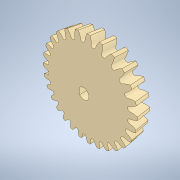
# Autodesk Inventor part: Шестерня мотора 2
Saved by Autodesk Inventor 2021.1 (Build 251245010, 245A)
## iProperties
Created: 2026-05-03
Part Number: Шестерня мотора 2
Material: Generic
Document SubType Name: Modeling
Designer: Андрей Тарасов
Density: 1 g/cm^3
Appearance: Default
Author: Андрей Тарасов
Autodesk Inventor part; units mm, degrees
ref_plane "YZ Plane" through (0, 0, 0) normal (1, 0, 0) x (0, 1, 0)
ref_plane "XZ Plane" through (0, 0, 0) normal (0, 1, 0) x (-1, 0, 0)
ref_plane "XY Plane" through (0, 0, 0) normal (0, 0, 1) x (1, 0, 0)
sketch "Sketch1" plane through (0, 0, 0) normal (0, 0, 1) x (1, 0, 0)
  spline S0 degree 3 poles (-1.8162, 21.8754) (-1.7746, 21.8042) (-1.6912, 21.6617) (-1.5738, 21.4438) (-1.4622, 21.2229) (-1.3577, 20.9985) (-1.2608, 20.7707) (-1.1726, 20.5395) (-1.094, 20.3047) (-1.0278, 20.0662) (-0.9752, 19.824) (-0.9571, 19.6181) (-0.9246, 19.4563) (-0.8956, 19.3359) (-0.8558, 19.2186) (-0.8088, 19.104) (-0.7488, 18.9955) (-0.6764, 18.8948) (-0.6025, 18.8222) (-0.5374, 18.7714) (-0.4841, 18.7397) (-0.4281, 18.7132) (-0.3698, 18.6922) (-0.3092, 18.6789) (-0.1857, 18.6689) (0, 18.6787) (0.1857, 18.6689) (0.3092, 18.6789) (0.3698, 18.6922) (0.4281, 18.7132) (0.4841, 18.7397) (0.5374, 18.7714) (0.6025, 18.8222) (0.6764, 18.8948) (0.7488, 18.9955) (0.8088, 19.104) (0.8558, 19.2186) (0.8956, 19.3359) (0.9246, 19.4563) (0.9571, 19.6181) (0.9752, 19.824) (1.0278, 20.0662) (1.094, 20.3047) (1.1726, 20.5395) (1.2608, 20.7707) (1.3577, 20.9985) (1.4622, 21.2229) (1.5738, 21.4438) (1.6912, 21.6617) (1.7746, 21.8042) (1.8162, 21.8754) knots 0 0 0 0 0.024749 0.049497 0.074246 0.098994 0.123742 0.14849 0.173237 0.197983 0.222726 0.247472 0.259846 0.272219 0.284591 0.296962 0.309334 0.321703 0.334061 0.340251 0.346439 0.35262 0.358805 0.364993 0.371173 0.39592 0.420667 0.426846 0.433034 0.439219 0.4454 0.451589 0.457778 0.470137 0.482506 0.494877 0.507248 0.51962 0.531993 0.544367 0.569113 0.593856 0.618602 0.643349 0.668097 0.692845 0.717593 0.742342 0.767091 0.791839 0.791839 0.791839 0.791839
  circle A0 centre (0, 0) radius 18.6744 construction
  circle A1 centre (0, 0) radius 19.7335 construction
  circle A2 centre (0, 0) radius 21 construction
  circle A3 centre (0, 0) radius 21.9506
  spline S1 degree 3 poles (-6.6384, 20.9228) (-6.5819, 20.8626) (-6.469, 20.7423) (-6.306, 20.556) (-6.1481, 20.3654) (-5.9963, 20.1699) (-5.8512, 19.9694) (-5.7136, 19.7636) (-5.5848, 19.5521) (-5.4672, 19.3344) (-5.362, 19.1099) (-5.2985, 18.9133) (-5.2309, 18.7627) (-5.1758, 18.6518) (-5.1109, 18.5464) (-5.0395, 18.4451) (-4.957, 18.3526) (-4.8639, 18.2705) (-4.7757, 18.2162) (-4.701, 18.1811) (-4.6419, 18.1621) (-4.5815, 18.1488) (-4.5199, 18.1413) (-4.4579, 18.1417) (-4.3352, 18.1595) (-4.1564, 18.2104) (-3.9732, 18.2422) (-3.855, 18.2794) (-3.7989, 18.3059) (-3.7467, 18.3393) (-3.698, 18.3775) (-3.6531, 18.4203) (-3.6009, 18.4843) (-3.5451, 18.5715) (-3.4968, 18.6859) (-3.4626, 18.805) (-3.4422, 18.9272) (-3.4295, 19.0504) (-3.428, 19.1742) (-3.4324, 19.3392) (-3.4605, 19.5439) (-3.4631, 19.7918) (-3.4516, 20.039) (-3.4273, 20.2854) (-3.3927, 20.5305) (-3.3489, 20.7742) (-3.297, 21.0162) (-3.2374, 21.2564) (-3.1714, 21.495) (-3.1218, 21.6524) (-3.0971, 21.7311) knots 0 0 0 0 0.024749 0.049497 0.074246 0.098994 0.123742 0.14849 0.173237 0.197983 0.222726 0.247472 0.259846 0.272219 0.284591 0.296962 0.309334 0.321703 0.334061 0.340251 0.346439 0.35262 0.358805 0.364993 0.371173 0.39592 0.420667 0.426846 0.433034 0.439219 0.4454 0.451589 0.457778 0.470137 0.482506 0.494877 0.507248 0.51962 0.531993 0.544367 0.569113 0.593856 0.618602 0.643349 0.668097 0.692845 0.717593 0.742342 0.767091 0.791839 0.791839 0.791839 0.791839
  spline S2 degree 3 poles (-11.1277, 18.921) (-11.0593, 18.8749) (-10.9224, 18.7828) (-10.7221, 18.6374) (-10.5257, 18.4867) (-10.3342, 18.3299) (-10.1481, 18.1667) (-9.9682, 17.9967) (-9.7956, 17.8192) (-9.6324, 17.6331) (-9.4799, 17.4376) (-9.3743, 17.2601) (-9.2748, 17.1283) (-9.1964, 17.0325) (-9.1097, 16.9441) (-9.0176, 16.8612) (-8.9165, 16.7894) (-8.8075, 16.7301) (-8.7095, 16.6967) (-8.6288, 16.6792) (-8.567, 16.6738) (-8.5051, 16.6743) (-8.4434, 16.6807) (-8.383, 16.6949) (-8.2674, 16.7395) (-8.1044, 16.829) (-7.9328, 16.9007) (-7.8259, 16.9632) (-7.7771, 17.0016) (-7.7336, 17.0458) (-7.6947, 17.0939) (-7.6604, 17.1456) (-7.6238, 17.2196) (-7.5887, 17.317) (-7.5672, 17.4393) (-7.5603, 17.563) (-7.5676, 17.6867) (-7.5826, 17.8096) (-7.6087, 17.9307) (-7.6497, 18.0906) (-7.7226, 18.2839) (-7.7804, 18.525) (-7.8242, 18.7686) (-7.8553, 19.0142) (-7.8761, 19.2608) (-7.8876, 19.5081) (-7.8908, 19.7556) (-7.8862, 20.0031) (-7.8749, 20.2504) (-7.8617, 20.4148) (-7.855, 20.4971) knots 0 0 0 0 0.024749 0.049497 0.074246 0.098994 0.123742 0.14849 0.173237 0.197983 0.222726 0.247472 0.259846 0.272219 0.284591 0.296962 0.309334 0.321703 0.334061 0.340251 0.346439 0.35262 0.358805 0.364993 0.371173 0.39592 0.420667 0.426846 0.433034 0.439219 0.4454 0.451589 0.457778 0.470137 0.482506 0.494877 0.507248 0.51962 0.531993 0.544367 0.569113 0.593856 0.618602 0.643349 0.668097 0.692845 0.717593 0.742342 0.767091 0.791839 0.791839 0.791839 0.791839
  spline S3 degree 3 poles (-15.059, 15.9705) (-14.9821, 15.9408) (-14.8281, 15.8814) (-14.6005, 15.7842) (-14.3755, 15.681) (-14.1539, 15.5708) (-13.9361, 15.4531) (-13.7229, 15.3273) (-13.5151, 15.1927) (-13.3146, 15.0476) (-13.1225, 14.8909) (-12.98, 14.7414) (-12.8537, 14.635) (-12.7559, 14.559) (-12.6517, 14.4922) (-12.5435, 14.4319) (-12.429, 14.3844) (-12.3095, 14.3508) (-12.2065, 14.3401) (-12.1239, 14.341) (-12.0625, 14.3494) (-12.0022, 14.3636) (-11.9435, 14.3836) (-11.8878, 14.4109) (-11.785, 14.4802) (-11.646, 14.6036) (-11.4947, 14.7117) (-11.4043, 14.7965) (-11.3653, 14.8447) (-11.3328, 14.8975) (-11.3055, 14.9531) (-11.2836, 15.0111) (-11.2644, 15.0914) (-11.2519, 15.1942) (-11.258, 15.3182) (-11.2788, 15.4404) (-11.3136, 15.5593) (-11.3555, 15.6758) (-11.4079, 15.788) (-11.4834, 15.9348) (-11.5976, 16.107) (-11.7075, 16.3292) (-11.8044, 16.557) (-11.8894, 16.7895) (-11.9646, 17.0253) (-12.0308, 17.2638) (-12.089, 17.5044) (-12.1396, 17.7467) (-12.1836, 17.9903) (-12.2073, 18.1536) (-12.2191, 18.2352) knots 0 0 0 0 0.024749 0.049497 0.074246 0.098994 0.123742 0.14849 0.173237 0.197983 0.222726 0.247472 0.259846 0.272219 0.284591 0.296962 0.309334 0.321703 0.334061 0.340251 0.346439 0.35262 0.358805 0.364993 0.371173 0.39592 0.420667 0.426846 0.433034 0.439219 0.4454 0.451589 0.457778 0.470137 0.482506 0.494877 0.507248 0.51962 0.531993 0.544367 0.569113 0.593856 0.618602 0.643349 0.668097 0.692845 0.717593 0.742342 0.767091 0.791839 0.791839 0.791839 0.791839
  spline S4 degree 3 poles (-18.2352, 12.2191) (-18.1536, 12.2073) (-17.9903, 12.1836) (-17.7467, 12.1396) (-17.5044, 12.089) (-17.2638, 12.0308) (-17.0253, 11.9646) (-16.7895, 11.8894) (-16.557, 11.8044) (-16.3292, 11.7075) (-16.107, 11.5976) (-15.9348, 11.4834) (-15.788, 11.4079) (-15.6758, 11.3555) (-15.5593, 11.3136) (-15.4404, 11.2788) (-15.3182, 11.258) (-15.1942, 11.2519) (-15.0914, 11.2644) (-15.0111, 11.2836) (-14.9531, 11.3055) (-14.8975, 11.3328) (-14.8447, 11.3653) (-14.7965, 11.4043) (-14.7117, 11.4947) (-14.6036, 11.646) (-14.4802, 11.785) (-14.4109, 11.8878) (-14.3836, 11.9435) (-14.3636, 12.0022) (-14.3494, 12.0625) (-14.341, 12.1239) (-14.3401, 12.2065) (-14.3508, 12.3095) (-14.3844, 12.429) (-14.4319, 12.5435) (-14.4922, 12.6517) (-14.559, 12.7559) (-14.635, 12.8537) (-14.7414, 12.98) (-14.8909, 13.1225) (-15.0476, 13.3146) (-15.1927, 13.5151) (-15.3273, 13.7229) (-15.4531, 13.9361) (-15.5708, 14.1539) (-15.681, 14.3755) (-15.7842, 14.6005) (-15.8814, 14.8281) (-15.9408, 14.9821) (-15.9705, 15.059) knots 0 0 0 0 0.024749 0.049497 0.074246 0.098994 0.123742 0.14849 0.173237 0.197983 0.222726 0.247472 0.259846 0.272219 0.284591 0.296962 0.309334 0.321703 0.334061 0.340251 0.346439 0.35262 0.358805 0.364993 0.371173 0.39592 0.420667 0.426846 0.433034 0.439219 0.4454 0.451589 0.457778 0.470137 0.482506 0.494877 0.507248 0.51962 0.531993 0.544367 0.569113 0.593856 0.618602 0.643349 0.668097 0.692845 0.717593 0.742342 0.767091 0.791839 0.791839 0.791839 0.791839
  spline S5 degree 3 poles (-20.4971, 7.855) (-20.4148, 7.8617) (-20.2504, 7.8749) (-20.0031, 7.8862) (-19.7556, 7.8908) (-19.5081, 7.8876) (-19.2608, 7.8761) (-19.0142, 7.8553) (-18.7686, 7.8242) (-18.525, 7.7804) (-18.2839, 7.7226) (-18.0906, 7.6497) (-17.9307, 7.6087) (-17.8096, 7.5826) (-17.6867, 7.5676) (-17.563, 7.5603) (-17.4393, 7.5672) (-17.317, 7.5887) (-17.2196, 7.6238) (-17.1456, 7.6604) (-17.0939, 7.6947) (-17.0458, 7.7336) (-17.0016, 7.7771) (-16.9632, 7.8259) (-16.9007, 7.9328) (-16.829, 8.1044) (-16.7395, 8.2674) (-16.6949, 8.383) (-16.6807, 8.4434) (-16.6743, 8.5051) (-16.6738, 8.567) (-16.6792, 8.6288) (-16.6967, 8.7095) (-16.7301, 8.8075) (-16.7894, 8.9165) (-16.8612, 9.0176) (-16.9441, 9.1097) (-17.0325, 9.1964) (-17.1283, 9.2748) (-17.2601, 9.3743) (-17.4376, 9.4799) (-17.6331, 9.6324) (-17.8192, 9.7956) (-17.9967, 9.9682) (-18.1667, 10.1481) (-18.3299, 10.3342) (-18.4867, 10.5257) (-18.6374, 10.7221) (-18.7828, 10.9224) (-18.8749, 11.0593) (-18.921, 11.1277) knots 0 0 0 0 0.024749 0.049497 0.074246 0.098994 0.123742 0.14849 0.173237 0.197983 0.222726 0.247472 0.259846 0.272219 0.284591 0.296962 0.309334 0.321703 0.334061 0.340251 0.346439 0.35262 0.358805 0.364993 0.371173 0.39592 0.420667 0.426846 0.433034 0.439219 0.4454 0.451589 0.457778 0.470137 0.482506 0.494877 0.507248 0.51962 0.531993 0.544367 0.569113 0.593856 0.618602 0.643349 0.668097 0.692845 0.717593 0.742342 0.767091 0.791839 0.791839 0.791839 0.791839
  spline S6 degree 3 poles (-21.7311, 3.0971) (-21.6524, 3.1218) (-21.495, 3.1714) (-21.2564, 3.2374) (-21.0162, 3.297) (-20.7742, 3.3489) (-20.5305, 3.3927) (-20.2854, 3.4273) (-20.039, 3.4516) (-19.7918, 3.4631) (-19.5439, 3.4605) (-19.3392, 3.4324) (-19.1742, 3.428) (-19.0504, 3.4295) (-18.9272, 3.4422) (-18.805, 3.4626) (-18.6859, 3.4968) (-18.5715, 3.5451) (-18.4843, 3.6009) (-18.4203, 3.6531) (-18.3775, 3.698) (-18.3393, 3.7467) (-18.3059, 3.7989) (-18.2794, 3.855) (-18.2422, 3.9732) (-18.2104, 4.1564) (-18.1595, 4.3352) (-18.1417, 4.4579) (-18.1413, 4.5199) (-18.1488, 4.5815) (-18.1621, 4.6419) (-18.1811, 4.701) (-18.2162, 4.7757) (-18.2705, 4.8639) (-18.3526, 4.957) (-18.4451, 5.0395) (-18.5464, 5.1109) (-18.6518, 5.1758) (-18.7627, 5.2309) (-18.9133, 5.2985) (-19.1099, 5.362) (-19.3344, 5.4672) (-19.5521, 5.5848) (-19.7636, 5.7136) (-19.9694, 5.8512) (-20.1699, 5.9963) (-20.3654, 6.1481) (-20.556, 6.306) (-20.7423, 6.469) (-20.8626, 6.5819) (-20.9228, 6.6384) knots 0 0 0 0 0.024749 0.049497 0.074246 0.098994 0.123742 0.14849 0.173237 0.197983 0.222726 0.247472 0.259846 0.272219 0.284591 0.296962 0.309334 0.321703 0.334061 0.340251 0.346439 0.35262 0.358805 0.364993 0.371173 0.39592 0.420667 0.426846 0.433034 0.439219 0.4454 0.451589 0.457778 0.470137 0.482506 0.494877 0.507248 0.51962 0.531993 0.544367 0.569113 0.593856 0.618602 0.643349 0.668097 0.692845 0.717593 0.742342 0.767091 0.791839 0.791839 0.791839 0.791839
  spline S7 degree 3 poles (-21.8754, -1.8162) (-21.8042, -1.7746) (-21.6617, -1.6912) (-21.4438, -1.5738) (-21.2229, -1.4622) (-20.9985, -1.3577) (-20.7707, -1.2608) (-20.5395, -1.1726) (-20.3047, -1.094) (-20.0662, -1.0278) (-19.824, -0.9752) (-19.6181, -0.9571) (-19.4563, -0.9246) (-19.3359, -0.8956) (-19.2186, -0.8558) (-19.104, -0.8088) (-18.9955, -0.7488) (-18.8948, -0.6764) (-18.8222, -0.6025) (-18.7714, -0.5374) (-18.7397, -0.4841) (-18.7132, -0.4281) (-18.6922, -0.3698) (-18.6789, -0.3092) (-18.6689, -0.1857) (-18.6787, 0) (-18.6689, 0.1857) (-18.6789, 0.3092) (-18.6922, 0.3698) (-18.7132, 0.4281) (-18.7397, 0.4841) (-18.7714, 0.5374) (-18.8222, 0.6025) (-18.8948, 0.6764) (-18.9955, 0.7488) (-19.104, 0.8088) (-19.2186, 0.8558) (-19.3359, 0.8956) (-19.4563, 0.9246) (-19.6181, 0.9571) (-19.824, 0.9752) (-20.0662, 1.0278) (-20.3047, 1.094) (-20.5395, 1.1726) (-20.7707, 1.2608) (-20.9985, 1.3577) (-21.2229, 1.4622) (-21.4438, 1.5738) (-21.6617, 1.6912) (-21.8042, 1.7746) (-21.8754, 1.8162) knots 0 0 0 0 0.024749 0.049497 0.074246 0.098994 0.123742 0.14849 0.173237 0.197983 0.222726 0.247472 0.259846 0.272219 0.284591 0.296962 0.309334 0.321703 0.334061 0.340251 0.346439 0.35262 0.358805 0.364993 0.371173 0.39592 0.420667 0.426846 0.433034 0.439219 0.4454 0.451589 0.457778 0.470137 0.482506 0.494877 0.507248 0.51962 0.531993 0.544367 0.569113 0.593856 0.618602 0.643349 0.668097 0.692845 0.717593 0.742342 0.767091 0.791839 0.791839 0.791839 0.791839
  spline S8 degree 3 poles (-20.9228, -6.6384) (-20.8626, -6.5819) (-20.7423, -6.469) (-20.556, -6.306) (-20.3654, -6.1481) (-20.1699, -5.9963) (-19.9694, -5.8512) (-19.7636, -5.7136) (-19.5521, -5.5848) (-19.3344, -5.4672) (-19.1099, -5.362) (-18.9133, -5.2985) (-18.7627, -5.2309) (-18.6518, -5.1758) (-18.5464, -5.1109) (-18.4451, -5.0395) (-18.3526, -4.957) (-18.2705, -4.8639) (-18.2162, -4.7757) (-18.1811, -4.701) (-18.1621, -4.6419) (-18.1488, -4.5815) (-18.1413, -4.5199) (-18.1417, -4.4579) (-18.1595, -4.3352) (-18.2104, -4.1564) (-18.2422, -3.9732) (-18.2794, -3.855) (-18.3059, -3.7989) (-18.3393, -3.7467) (-18.3775, -3.698) (-18.4203, -3.6531) (-18.4843, -3.6009) (-18.5715, -3.5451) (-18.6859, -3.4968) (-18.805, -3.4626) (-18.9272, -3.4422) (-19.0504, -3.4295) (-19.1742, -3.428) (-19.3392, -3.4324) (-19.5439, -3.4605) (-19.7918, -3.4631) (-20.039, -3.4516) (-20.2854, -3.4273) (-20.5305, -3.3927) (-20.7742, -3.3489) (-21.0162, -3.297) (-21.2564, -3.2374) (-21.495, -3.1714) (-21.6524, -3.1218) (-21.7311, -3.0971) knots 0 0 0 0 0.024749 0.049497 0.074246 0.098994 0.123742 0.14849 0.173237 0.197983 0.222726 0.247472 0.259846 0.272219 0.284591 0.296962 0.309334 0.321703 0.334061 0.340251 0.346439 0.35262 0.358805 0.364993 0.371173 0.39592 0.420667 0.426846 0.433034 0.439219 0.4454 0.451589 0.457778 0.470137 0.482506 0.494877 0.507248 0.51962 0.531993 0.544367 0.569113 0.593856 0.618602 0.643349 0.668097 0.692845 0.717593 0.742342 0.767091 0.791839 0.791839 0.791839 0.791839
  spline S9 degree 3 poles (-18.921, -11.1277) (-18.8749, -11.0593) (-18.7828, -10.9224) (-18.6374, -10.7221) (-18.4867, -10.5257) (-18.3299, -10.3342) (-18.1667, -10.1481) (-17.9967, -9.9682) (-17.8192, -9.7956) (-17.6331, -9.6324) (-17.4376, -9.4799) (-17.2601, -9.3743) (-17.1283, -9.2748) (-17.0325, -9.1964) (-16.9441, -9.1097) (-16.8612, -9.0176) (-16.7894, -8.9165) (-16.7301, -8.8075) (-16.6967, -8.7095) (-16.6792, -8.6288) (-16.6738, -8.567) (-16.6743, -8.5051) (-16.6807, -8.4434) (-16.6949, -8.383) (-16.7395, -8.2674) (-16.829, -8.1044) (-16.9007, -7.9328) (-16.9632, -7.8259) (-17.0016, -7.7771) (-17.0458, -7.7336) (-17.0939, -7.6947) (-17.1456, -7.6604) (-17.2196, -7.6238) (-17.317, -7.5887) (-17.4393, -7.5672) (-17.563, -7.5603) (-17.6867, -7.5676) (-17.8096, -7.5826) (-17.9307, -7.6087) (-18.0906, -7.6497) (-18.2839, -7.7226) (-18.525, -7.7804) (-18.7686, -7.8242) (-19.0142, -7.8553) (-19.2608, -7.8761) (-19.5081, -7.8876) (-19.7556, -7.8908) (-20.0031, -7.8862) (-20.2504, -7.8749) (-20.4148, -7.8617) (-20.4971, -7.855) knots 0 0 0 0 0.024749 0.049497 0.074246 0.098994 0.123742 0.14849 0.173237 0.197983 0.222726 0.247472 0.259846 0.272219 0.284591 0.296962 0.309334 0.321703 0.334061 0.340251 0.346439 0.35262 0.358805 0.364993 0.371173 0.39592 0.420667 0.426846 0.433034 0.439219 0.4454 0.451589 0.457778 0.470137 0.482506 0.494877 0.507248 0.51962 0.531993 0.544367 0.569113 0.593856 0.618602 0.643349 0.668097 0.692845 0.717593 0.742342 0.767091 0.791839 0.791839 0.791839 0.791839
  spline S10 degree 3 poles (-15.9705, -15.059) (-15.9408, -14.9821) (-15.8814, -14.8281) (-15.7842, -14.6005) (-15.681, -14.3755) (-15.5708, -14.1539) (-15.4531, -13.9361) (-15.3273, -13.7229) (-15.1927, -13.5151) (-15.0476, -13.3146) (-14.8909, -13.1225) (-14.7414, -12.98) (-14.635, -12.8537) (-14.559, -12.7559) (-14.4922, -12.6517) (-14.4319, -12.5435) (-14.3844, -12.429) (-14.3508, -12.3095) (-14.3401, -12.2065) (-14.341, -12.1239) (-14.3494, -12.0625) (-14.3636, -12.0022) (-14.3836, -11.9435) (-14.4109, -11.8878) (-14.4802, -11.785) (-14.6036, -11.646) (-14.7117, -11.4947) (-14.7965, -11.4043) (-14.8447, -11.3653) (-14.8975, -11.3328) (-14.9531, -11.3055) (-15.0111, -11.2836) (-15.0914, -11.2644) (-15.1942, -11.2519) (-15.3182, -11.258) (-15.4404, -11.2788) (-15.5593, -11.3136) (-15.6758, -11.3555) (-15.788, -11.4079) (-15.9348, -11.4834) (-16.107, -11.5976) (-16.3292, -11.7075) (-16.557, -11.8044) (-16.7895, -11.8894) (-17.0253, -11.9646) (-17.2638, -12.0308) (-17.5044, -12.089) (-17.7467, -12.1396) (-17.9903, -12.1836) (-18.1536, -12.2073) (-18.2352, -12.2191) knots 0 0 0 0 0.024749 0.049497 0.074246 0.098994 0.123742 0.14849 0.173237 0.197983 0.222726 0.247472 0.259846 0.272219 0.284591 0.296962 0.309334 0.321703 0.334061 0.340251 0.346439 0.35262 0.358805 0.364993 0.371173 0.39592 0.420667 0.426846 0.433034 0.439219 0.4454 0.451589 0.457778 0.470137 0.482506 0.494877 0.507248 0.51962 0.531993 0.544367 0.569113 0.593856 0.618602 0.643349 0.668097 0.692845 0.717593 0.742342 0.767091 0.791839 0.791839 0.791839 0.791839
  spline S11 degree 3 poles (-12.2191, -18.2352) (-12.2073, -18.1536) (-12.1836, -17.9903) (-12.1396, -17.7467) (-12.089, -17.5044) (-12.0308, -17.2638) (-11.9646, -17.0253) (-11.8894, -16.7895) (-11.8044, -16.557) (-11.7075, -16.3292) (-11.5976, -16.107) (-11.4834, -15.9348) (-11.4079, -15.788) (-11.3555, -15.6758) (-11.3136, -15.5593) (-11.2788, -15.4404) (-11.258, -15.3182) (-11.2519, -15.1942) (-11.2644, -15.0914) (-11.2836, -15.0111) (-11.3055, -14.9531) (-11.3328, -14.8975) (-11.3653, -14.8447) (-11.4043, -14.7965) (-11.4947, -14.7117) (-11.646, -14.6036) (-11.785, -14.4802) (-11.8878, -14.4109) (-11.9435, -14.3836) (-12.0022, -14.3636) (-12.0625, -14.3494) (-12.1239, -14.341) (-12.2065, -14.3401) (-12.3095, -14.3508) (-12.429, -14.3844) (-12.5435, -14.4319) (-12.6517, -14.4922) (-12.7559, -14.559) (-12.8537, -14.635) (-12.98, -14.7414) (-13.1225, -14.8909) (-13.3146, -15.0476) (-13.5151, -15.1927) (-13.7229, -15.3273) (-13.9361, -15.4531) (-14.1539, -15.5708) (-14.3755, -15.681) (-14.6005, -15.7842) (-14.8281, -15.8814) (-14.9821, -15.9408) (-15.059, -15.9705) knots 0 0 0 0 0.024749 0.049497 0.074246 0.098994 0.123742 0.14849 0.173237 0.197983 0.222726 0.247472 0.259846 0.272219 0.284591 0.296962 0.309334 0.321703 0.334061 0.340251 0.346439 0.35262 0.358805 0.364993 0.371173 0.39592 0.420667 0.426846 0.433034 0.439219 0.4454 0.451589 0.457778 0.470137 0.482506 0.494877 0.507248 0.51962 0.531993 0.544367 0.569113 0.593856 0.618602 0.643349 0.668097 0.692845 0.717593 0.742342 0.767091 0.791839 0.791839 0.791839 0.791839
  spline S12 degree 3 poles (-7.855, -20.4971) (-7.8617, -20.4148) (-7.8749, -20.2504) (-7.8862, -20.0031) (-7.8908, -19.7556) (-7.8876, -19.5081) (-7.8761, -19.2608) (-7.8553, -19.0142) (-7.8242, -18.7686) (-7.7804, -18.525) (-7.7226, -18.2839) (-7.6497, -18.0906) (-7.6087, -17.9307) (-7.5826, -17.8096) (-7.5676, -17.6867) (-7.5603, -17.563) (-7.5672, -17.4393) (-7.5887, -17.317) (-7.6238, -17.2196) (-7.6604, -17.1456) (-7.6947, -17.0939) (-7.7336, -17.0458) (-7.7771, -17.0016) (-7.8259, -16.9632) (-7.9328, -16.9007) (-8.1044, -16.829) (-8.2674, -16.7395) (-8.383, -16.6949) (-8.4434, -16.6807) (-8.5051, -16.6743) (-8.567, -16.6738) (-8.6288, -16.6792) (-8.7095, -16.6967) (-8.8075, -16.7301) (-8.9165, -16.7894) (-9.0176, -16.8612) (-9.1097, -16.9441) (-9.1964, -17.0325) (-9.2748, -17.1283) (-9.3743, -17.2601) (-9.4799, -17.4376) (-9.6324, -17.6331) (-9.7956, -17.8192) (-9.9682, -17.9967) (-10.1481, -18.1667) (-10.3342, -18.3299) (-10.5257, -18.4867) (-10.7221, -18.6374) (-10.9224, -18.7828) (-11.0593, -18.8749) (-11.1277, -18.921) knots 0 0 0 0 0.024749 0.049497 0.074246 0.098994 0.123742 0.14849 0.173237 0.197983 0.222726 0.247472 0.259846 0.272219 0.284591 0.296962 0.309334 0.321703 0.334061 0.340251 0.346439 0.35262 0.358805 0.364993 0.371173 0.39592 0.420667 0.426846 0.433034 0.439219 0.4454 0.451589 0.457778 0.470137 0.482506 0.494877 0.507248 0.51962 0.531993 0.544367 0.569113 0.593856 0.618602 0.643349 0.668097 0.692845 0.717593 0.742342 0.767091 0.791839 0.791839 0.791839 0.791839
  spline S13 degree 3 poles (-3.0971, -21.7311) (-3.1218, -21.6524) (-3.1714, -21.495) (-3.2374, -21.2564) (-3.297, -21.0162) (-3.3489, -20.7742) (-3.3927, -20.5305) (-3.4273, -20.2854) (-3.4516, -20.039) (-3.4631, -19.7918) (-3.4605, -19.5439) (-3.4324, -19.3392) (-3.428, -19.1742) (-3.4295, -19.0504) (-3.4422, -18.9272) (-3.4626, -18.805) (-3.4968, -18.6859) (-3.5451, -18.5715) (-3.6009, -18.4843) (-3.6531, -18.4203) (-3.698, -18.3775) (-3.7467, -18.3393) (-3.7989, -18.3059) (-3.855, -18.2794) (-3.9732, -18.2422) (-4.1564, -18.2104) (-4.3352, -18.1595) (-4.4579, -18.1417) (-4.5199, -18.1413) (-4.5815, -18.1488) (-4.6419, -18.1621) (-4.701, -18.1811) (-4.7757, -18.2162) (-4.8639, -18.2705) (-4.957, -18.3526) (-5.0395, -18.4451) (-5.1109, -18.5464) (-5.1758, -18.6518) (-5.2309, -18.7627) (-5.2985, -18.9133) (-5.362, -19.1099) (-5.4672, -19.3344) (-5.5848, -19.5521) (-5.7136, -19.7636) (-5.8512, -19.9694) (-5.9963, -20.1699) (-6.1481, -20.3654) (-6.306, -20.556) (-6.469, -20.7423) (-6.5819, -20.8626) (-6.6384, -20.9228) knots 0 0 0 0 0.024749 0.049497 0.074246 0.098994 0.123742 0.14849 0.173237 0.197983 0.222726 0.247472 0.259846 0.272219 0.284591 0.296962 0.309334 0.321703 0.334061 0.340251 0.346439 0.35262 0.358805 0.364993 0.371173 0.39592 0.420667 0.426846 0.433034 0.439219 0.4454 0.451589 0.457778 0.470137 0.482506 0.494877 0.507248 0.51962 0.531993 0.544367 0.569113 0.593856 0.618602 0.643349 0.668097 0.692845 0.717593 0.742342 0.767091 0.791839 0.791839 0.791839 0.791839
  spline S14 degree 3 poles (1.8162, -21.8754) (1.7746, -21.8042) (1.6912, -21.6617) (1.5738, -21.4438) (1.4622, -21.2229) (1.3577, -20.9985) (1.2608, -20.7707) (1.1726, -20.5395) (1.094, -20.3047) (1.0278, -20.0662) (0.9752, -19.824) (0.9571, -19.6181) (0.9246, -19.4563) (0.8956, -19.3359) (0.8558, -19.2186) (0.8088, -19.104) (0.7488, -18.9955) (0.6764, -18.8948) (0.6025, -18.8222) (0.5374, -18.7714) (0.4841, -18.7397) (0.4281, -18.7132) (0.3698, -18.6922) (0.3092, -18.6789) (0.1857, -18.6689) (0, -18.6787) (-0.1857, -18.6689) (-0.3092, -18.6789) (-0.3698, -18.6922) (-0.4281, -18.7132) (-0.4841, -18.7397) (-0.5374, -18.7714) (-0.6025, -18.8222) (-0.6764, -18.8948) (-0.7488, -18.9955) (-0.8088, -19.104) (-0.8558, -19.2186) (-0.8956, -19.3359) (-0.9246, -19.4563) (-0.9571, -19.6181) (-0.9752, -19.824) (-1.0278, -20.0662) (-1.094, -20.3047) (-1.1726, -20.5395) (-1.2608, -20.7707) (-1.3577, -20.9985) (-1.4622, -21.2229) (-1.5738, -21.4438) (-1.6912, -21.6617) (-1.7746, -21.8042) (-1.8162, -21.8754) knots 0 0 0 0 0.024749 0.049497 0.074246 0.098994 0.123742 0.14849 0.173237 0.197983 0.222726 0.247472 0.259846 0.272219 0.284591 0.296962 0.309334 0.321703 0.334061 0.340251 0.346439 0.35262 0.358805 0.364993 0.371173 0.39592 0.420667 0.426846 0.433034 0.439219 0.4454 0.451589 0.457778 0.470137 0.482506 0.494877 0.507248 0.51962 0.531993 0.544367 0.569113 0.593856 0.618602 0.643349 0.668097 0.692845 0.717593 0.742342 0.767091 0.791839 0.791839 0.791839 0.791839
  spline S15 degree 3 poles (6.6384, -20.9228) (6.5819, -20.8626) (6.469, -20.7423) (6.306, -20.556) (6.1481, -20.3654) (5.9963, -20.1699) (5.8512, -19.9694) (5.7136, -19.7636) (5.5848, -19.5521) (5.4672, -19.3344) (5.362, -19.1099) (5.2985, -18.9133) (5.2309, -18.7627) (5.1758, -18.6518) (5.1109, -18.5464) (5.0395, -18.4451) (4.957, -18.3526) (4.8639, -18.2705) (4.7757, -18.2162) (4.701, -18.1811) (4.6419, -18.1621) (4.5815, -18.1488) (4.5199, -18.1413) (4.4579, -18.1417) (4.3352, -18.1595) (4.1564, -18.2104) (3.9732, -18.2422) (3.855, -18.2794) (3.7989, -18.3059) (3.7467, -18.3393) (3.698, -18.3775) (3.6531, -18.4203) (3.6009, -18.4843) (3.5451, -18.5715) (3.4968, -18.6859) (3.4626, -18.805) (3.4422, -18.9272) (3.4295, -19.0504) (3.428, -19.1742) (3.4324, -19.3392) (3.4605, -19.5439) (3.4631, -19.7918) (3.4516, -20.039) (3.4273, -20.2854) (3.3927, -20.5305) (3.3489, -20.7742) (3.297, -21.0162) (3.2374, -21.2564) (3.1714, -21.495) (3.1218, -21.6524) (3.0971, -21.7311) knots 0 0 0 0 0.024749 0.049497 0.074246 0.098994 0.123742 0.14849 0.173237 0.197983 0.222726 0.247472 0.259846 0.272219 0.284591 0.296962 0.309334 0.321703 0.334061 0.340251 0.346439 0.35262 0.358805 0.364993 0.371173 0.39592 0.420667 0.426846 0.433034 0.439219 0.4454 0.451589 0.457778 0.470137 0.482506 0.494877 0.507248 0.51962 0.531993 0.544367 0.569113 0.593856 0.618602 0.643349 0.668097 0.692845 0.717593 0.742342 0.767091 0.791839 0.791839 0.791839 0.791839
  spline S16 degree 3 poles (11.1277, -18.921) (11.0593, -18.8749) (10.9224, -18.7828) (10.7221, -18.6374) (10.5257, -18.4867) (10.3342, -18.3299) (10.1481, -18.1667) (9.9682, -17.9967) (9.7956, -17.8192) (9.6324, -17.6331) (9.4799, -17.4376) (9.3743, -17.2601) (9.2748, -17.1283) (9.1964, -17.0325) (9.1097, -16.9441) (9.0176, -16.8612) (8.9165, -16.7894) (8.8075, -16.7301) (8.7095, -16.6967) (8.6288, -16.6792) (8.567, -16.6738) (8.5051, -16.6743) (8.4434, -16.6807) (8.383, -16.6949) (8.2674, -16.7395) (8.1044, -16.829) (7.9328, -16.9007) (7.8259, -16.9632) (7.7771, -17.0016) (7.7336, -17.0458) (7.6947, -17.0939) (7.6604, -17.1456) (7.6238, -17.2196) (7.5887, -17.317) (7.5672, -17.4393) (7.5603, -17.563) (7.5676, -17.6867) (7.5826, -17.8096) (7.6087, -17.9307) (7.6497, -18.0906) (7.7226, -18.2839) (7.7804, -18.525) (7.8242, -18.7686) (7.8553, -19.0142) (7.8761, -19.2608) (7.8876, -19.5081) (7.8908, -19.7556) (7.8862, -20.0031) (7.8749, -20.2504) (7.8617, -20.4148) (7.855, -20.4971) knots 0 0 0 0 0.024749 0.049497 0.074246 0.098994 0.123742 0.14849 0.173237 0.197983 0.222726 0.247472 0.259846 0.272219 0.284591 0.296962 0.309334 0.321703 0.334061 0.340251 0.346439 0.35262 0.358805 0.364993 0.371173 0.39592 0.420667 0.426846 0.433034 0.439219 0.4454 0.451589 0.457778 0.470137 0.482506 0.494877 0.507248 0.51962 0.531993 0.544367 0.569113 0.593856 0.618602 0.643349 0.668097 0.692845 0.717593 0.742342 0.767091 0.791839 0.791839 0.791839 0.791839
  spline S17 degree 3 poles (15.059, -15.9705) (14.9821, -15.9408) (14.8281, -15.8814) (14.6005, -15.7842) (14.3755, -15.681) (14.1539, -15.5708) (13.9361, -15.4531) (13.7229, -15.3273) (13.5151, -15.1927) (13.3146, -15.0476) (13.1225, -14.8909) (12.98, -14.7414) (12.8537, -14.635) (12.7559, -14.559) (12.6517, -14.4922) (12.5435, -14.4319) (12.429, -14.3844) (12.3095, -14.3508) (12.2065, -14.3401) (12.1239, -14.341) (12.0625, -14.3494) (12.0022, -14.3636) (11.9435, -14.3836) (11.8878, -14.4109) (11.785, -14.4802) (11.646, -14.6036) (11.4947, -14.7117) (11.4043, -14.7965) (11.3653, -14.8447) (11.3328, -14.8975) (11.3055, -14.9531) (11.2836, -15.0111) (11.2644, -15.0914) (11.2519, -15.1942) (11.258, -15.3182) (11.2788, -15.4404) (11.3136, -15.5593) (11.3555, -15.6758) (11.4079, -15.788) (11.4834, -15.9348) (11.5976, -16.107) (11.7075, -16.3292) (11.8044, -16.557) (11.8894, -16.7895) (11.9646, -17.0253) (12.0308, -17.2638) (12.089, -17.5044) (12.1396, -17.7467) (12.1836, -17.9903) (12.2073, -18.1536) (12.2191, -18.2352) knots 0 0 0 0 0.024749 0.049497 0.074246 0.098994 0.123742 0.14849 0.173237 0.197983 0.222726 0.247472 0.259846 0.272219 0.284591 0.296962 0.309334 0.321703 0.334061 0.340251 0.346439 0.35262 0.358805 0.364993 0.371173 0.39592 0.420667 0.426846 0.433034 0.439219 0.4454 0.451589 0.457778 0.470137 0.482506 0.494877 0.507248 0.51962 0.531993 0.544367 0.569113 0.593856 0.618602 0.643349 0.668097 0.692845 0.717593 0.742342 0.767091 0.791839 0.791839 0.791839 0.791839
  spline S18 degree 3 poles (18.2352, -12.2191) (18.1536, -12.2073) (17.9903, -12.1836) (17.7467, -12.1396) (17.5044, -12.089) (17.2638, -12.0308) (17.0253, -11.9646) (16.7895, -11.8894) (16.557, -11.8044) (16.3292, -11.7075) (16.107, -11.5976) (15.9348, -11.4834) (15.788, -11.4079) (15.6758, -11.3555) (15.5593, -11.3136) (15.4404, -11.2788) (15.3182, -11.258) (15.1942, -11.2519) (15.0914, -11.2644) (15.0111, -11.2836) (14.9531, -11.3055) (14.8975, -11.3328) (14.8447, -11.3653) (14.7965, -11.4043) (14.7117, -11.4947) (14.6036, -11.646) (14.4802, -11.785) (14.4109, -11.8878) (14.3836, -11.9435) (14.3636, -12.0022) (14.3494, -12.0625) (14.341, -12.1239) (14.3401, -12.2065) (14.3508, -12.3095) (14.3844, -12.429) (14.4319, -12.5435) (14.4922, -12.6517) (14.559, -12.7559) (14.635, -12.8537) (14.7414, -12.98) (14.8909, -13.1225) (15.0476, -13.3146) (15.1927, -13.5151) (15.3273, -13.7229) (15.4531, -13.9361) (15.5708, -14.1539) (15.681, -14.3755) (15.7842, -14.6005) (15.8814, -14.8281) (15.9408, -14.9821) (15.9705, -15.059) knots 0 0 0 0 0.024749 0.049497 0.074246 0.098994 0.123742 0.14849 0.173237 0.197983 0.222726 0.247472 0.259846 0.272219 0.284591 0.296962 0.309334 0.321703 0.334061 0.340251 0.346439 0.35262 0.358805 0.364993 0.371173 0.39592 0.420667 0.426846 0.433034 0.439219 0.4454 0.451589 0.457778 0.470137 0.482506 0.494877 0.507248 0.51962 0.531993 0.544367 0.569113 0.593856 0.618602 0.643349 0.668097 0.692845 0.717593 0.742342 0.767091 0.791839 0.791839 0.791839 0.791839
  spline S19 degree 3 poles (20.4971, -7.855) (20.4148, -7.8617) (20.2504, -7.8749) (20.0031, -7.8862) (19.7556, -7.8908) (19.5081, -7.8876) (19.2608, -7.8761) (19.0142, -7.8553) (18.7686, -7.8242) (18.525, -7.7804) (18.2839, -7.7226) (18.0906, -7.6497) (17.9307, -7.6087) (17.8096, -7.5826) (17.6867, -7.5676) (17.563, -7.5603) (17.4393, -7.5672) (17.317, -7.5887) (17.2196, -7.6238) (17.1456, -7.6604) (17.0939, -7.6947) (17.0458, -7.7336) (17.0016, -7.7771) (16.9632, -7.8259) (16.9007, -7.9328) (16.829, -8.1044) (16.7395, -8.2674) (16.6949, -8.383) (16.6807, -8.4434) (16.6743, -8.5051) (16.6738, -8.567) (16.6792, -8.6288) (16.6967, -8.7095) (16.7301, -8.8075) (16.7894, -8.9165) (16.8612, -9.0176) (16.9441, -9.1097) (17.0325, -9.1964) (17.1283, -9.2748) (17.2601, -9.3743) (17.4376, -9.4799) (17.6331, -9.6324) (17.8192, -9.7956) (17.9967, -9.9682) (18.1667, -10.1481) (18.3299, -10.3342) (18.4867, -10.5257) (18.6374, -10.7221) (18.7828, -10.9224) (18.8749, -11.0593) (18.921, -11.1277) knots 0 0 0 0 0.024749 0.049497 0.074246 0.098994 0.123742 0.14849 0.173237 0.197983 0.222726 0.247472 0.259846 0.272219 0.284591 0.296962 0.309334 0.321703 0.334061 0.340251 0.346439 0.35262 0.358805 0.364993 0.371173 0.39592 0.420667 0.426846 0.433034 0.439219 0.4454 0.451589 0.457778 0.470137 0.482506 0.494877 0.507248 0.51962 0.531993 0.544367 0.569113 0.593856 0.618602 0.643349 0.668097 0.692845 0.717593 0.742342 0.767091 0.791839 0.791839 0.791839 0.791839
  spline S20 degree 3 poles (21.7311, -3.0971) (21.6524, -3.1218) (21.495, -3.1714) (21.2564, -3.2374) (21.0162, -3.297) (20.7742, -3.3489) (20.5305, -3.3927) (20.2854, -3.4273) (20.039, -3.4516) (19.7918, -3.4631) (19.5439, -3.4605) (19.3392, -3.4324) (19.1742, -3.428) (19.0504, -3.4295) (18.9272, -3.4422) (18.805, -3.4626) (18.6859, -3.4968) (18.5715, -3.5451) (18.4843, -3.6009) (18.4203, -3.6531) (18.3775, -3.698) (18.3393, -3.7467) (18.3059, -3.7989) (18.2794, -3.855) (18.2422, -3.9732) (18.2104, -4.1564) (18.1595, -4.3352) (18.1417, -4.4579) (18.1413, -4.5199) (18.1488, -4.5815) (18.1621, -4.6419) (18.1811, -4.701) (18.2162, -4.7757) (18.2705, -4.8639) (18.3526, -4.957) (18.4451, -5.0395) (18.5464, -5.1109) (18.6518, -5.1758) (18.7627, -5.2309) (18.9133, -5.2985) (19.1099, -5.362) (19.3344, -5.4672) (19.5521, -5.5848) (19.7636, -5.7136) (19.9694, -5.8512) (20.1699, -5.9963) (20.3654, -6.1481) (20.556, -6.306) (20.7423, -6.469) (20.8626, -6.5819) (20.9228, -6.6384) knots 0 0 0 0 0.024749 0.049497 0.074246 0.098994 0.123742 0.14849 0.173237 0.197983 0.222726 0.247472 0.259846 0.272219 0.284591 0.296962 0.309334 0.321703 0.334061 0.340251 0.346439 0.35262 0.358805 0.364993 0.371173 0.39592 0.420667 0.426846 0.433034 0.439219 0.4454 0.451589 0.457778 0.470137 0.482506 0.494877 0.507248 0.51962 0.531993 0.544367 0.569113 0.593856 0.618602 0.643349 0.668097 0.692845 0.717593 0.742342 0.767091 0.791839 0.791839 0.791839 0.791839
  spline S21 degree 3 poles (21.8754, 1.8162) (21.8042, 1.7746) (21.6617, 1.6912) (21.4438, 1.5738) (21.2229, 1.4622) (20.9985, 1.3577) (20.7707, 1.2608) (20.5395, 1.1726) (20.3047, 1.094) (20.0662, 1.0278) (19.824, 0.9752) (19.6181, 0.9571) (19.4563, 0.9246) (19.3359, 0.8956) (19.2186, 0.8558) (19.104, 0.8088) (18.9955, 0.7488) (18.8948, 0.6764) (18.8222, 0.6025) (18.7714, 0.5374) (18.7397, 0.4841) (18.7132, 0.4281) (18.6922, 0.3698) (18.6789, 0.3092) (18.6689, 0.1857) (18.6787, 0) (18.6689, -0.1857) (18.6789, -0.3092) (18.6922, -0.3698) (18.7132, -0.4281) (18.7397, -0.4841) (18.7714, -0.5374) (18.8222, -0.6025) (18.8948, -0.6764) (18.9955, -0.7488) (19.104, -0.8088) (19.2186, -0.8558) (19.3359, -0.8956) (19.4563, -0.9246) (19.6181, -0.9571) (19.824, -0.9752) (20.0662, -1.0278) (20.3047, -1.094) (20.5395, -1.1726) (20.7707, -1.2608) (20.9985, -1.3577) (21.2229, -1.4622) (21.4438, -1.5738) (21.6617, -1.6912) (21.8042, -1.7746) (21.8754, -1.8162) knots 0 0 0 0 0.024749 0.049497 0.074246 0.098994 0.123742 0.14849 0.173237 0.197983 0.222726 0.247472 0.259846 0.272219 0.284591 0.296962 0.309334 0.321703 0.334061 0.340251 0.346439 0.35262 0.358805 0.364993 0.371173 0.39592 0.420667 0.426846 0.433034 0.439219 0.4454 0.451589 0.457778 0.470137 0.482506 0.494877 0.507248 0.51962 0.531993 0.544367 0.569113 0.593856 0.618602 0.643349 0.668097 0.692845 0.717593 0.742342 0.767091 0.791839 0.791839 0.791839 0.791839
  spline S22 degree 3 poles (20.9228, 6.6384) (20.8626, 6.5819) (20.7423, 6.469) (20.556, 6.306) (20.3654, 6.1481) (20.1699, 5.9963) (19.9694, 5.8512) (19.7636, 5.7136) (19.5521, 5.5848) (19.3344, 5.4672) (19.1099, 5.362) (18.9133, 5.2985) (18.7627, 5.2309) (18.6518, 5.1758) (18.5464, 5.1109) (18.4451, 5.0395) (18.3526, 4.957) (18.2705, 4.8639) (18.2162, 4.7757) (18.1811, 4.701) (18.1621, 4.6419) (18.1488, 4.5815) (18.1413, 4.5199) (18.1417, 4.4579) (18.1595, 4.3352) (18.2104, 4.1564) (18.2422, 3.9732) (18.2794, 3.855) (18.3059, 3.7989) (18.3393, 3.7467) (18.3775, 3.698) (18.4203, 3.6531) (18.4843, 3.6009) (18.5715, 3.5451) (18.6859, 3.4968) (18.805, 3.4626) (18.9272, 3.4422) (19.0504, 3.4295) (19.1742, 3.428) (19.3392, 3.4324) (19.5439, 3.4605) (19.7918, 3.4631) (20.039, 3.4516) (20.2854, 3.4273) (20.5305, 3.3927) (20.7742, 3.3489) (21.0162, 3.297) (21.2564, 3.2374) (21.495, 3.1714) (21.6524, 3.1218) (21.7311, 3.0971) knots 0 0 0 0 0.024749 0.049497 0.074246 0.098994 0.123742 0.14849 0.173237 0.197983 0.222726 0.247472 0.259846 0.272219 0.284591 0.296962 0.309334 0.321703 0.334061 0.340251 0.346439 0.35262 0.358805 0.364993 0.371173 0.39592 0.420667 0.426846 0.433034 0.439219 0.4454 0.451589 0.457778 0.470137 0.482506 0.494877 0.507248 0.51962 0.531993 0.544367 0.569113 0.593856 0.618602 0.643349 0.668097 0.692845 0.717593 0.742342 0.767091 0.791839 0.791839 0.791839 0.791839
  spline S23 degree 3 poles (18.921, 11.1277) (18.8749, 11.0593) (18.7828, 10.9224) (18.6374, 10.7221) (18.4867, 10.5257) (18.3299, 10.3342) (18.1667, 10.1481) (17.9967, 9.9682) (17.8192, 9.7956) (17.6331, 9.6324) (17.4376, 9.4799) (17.2601, 9.3743) (17.1283, 9.2748) (17.0325, 9.1964) (16.9441, 9.1097) (16.8612, 9.0176) (16.7894, 8.9165) (16.7301, 8.8075) (16.6967, 8.7095) (16.6792, 8.6288) (16.6738, 8.567) (16.6743, 8.5051) (16.6807, 8.4434) (16.6949, 8.383) (16.7395, 8.2674) (16.829, 8.1044) (16.9007, 7.9328) (16.9632, 7.8259) (17.0016, 7.7771) (17.0458, 7.7336) (17.0939, 7.6947) (17.1456, 7.6604) (17.2196, 7.6238) (17.317, 7.5887) (17.4393, 7.5672) (17.563, 7.5603) (17.6867, 7.5676) (17.8096, 7.5826) (17.9307, 7.6087) (18.0906, 7.6497) (18.2839, 7.7226) (18.525, 7.7804) (18.7686, 7.8242) (19.0142, 7.8553) (19.2608, 7.8761) (19.5081, 7.8876) (19.7556, 7.8908) (20.0031, 7.8862) (20.2504, 7.8749) (20.4148, 7.8617) (20.4971, 7.855) knots 0 0 0 0 0.024749 0.049497 0.074246 0.098994 0.123742 0.14849 0.173237 0.197983 0.222726 0.247472 0.259846 0.272219 0.284591 0.296962 0.309334 0.321703 0.334061 0.340251 0.346439 0.35262 0.358805 0.364993 0.371173 0.39592 0.420667 0.426846 0.433034 0.439219 0.4454 0.451589 0.457778 0.470137 0.482506 0.494877 0.507248 0.51962 0.531993 0.544367 0.569113 0.593856 0.618602 0.643349 0.668097 0.692845 0.717593 0.742342 0.767091 0.791839 0.791839 0.791839 0.791839
  spline S24 degree 3 poles (15.9705, 15.059) (15.9408, 14.9821) (15.8814, 14.8281) (15.7842, 14.6005) (15.681, 14.3755) (15.5708, 14.1539) (15.4531, 13.9361) (15.3273, 13.7229) (15.1927, 13.5151) (15.0476, 13.3146) (14.8909, 13.1225) (14.7414, 12.98) (14.635, 12.8537) (14.559, 12.7559) (14.4922, 12.6517) (14.4319, 12.5435) (14.3844, 12.429) (14.3508, 12.3095) (14.3401, 12.2065) (14.341, 12.1239) (14.3494, 12.0625) (14.3636, 12.0022) (14.3836, 11.9435) (14.4109, 11.8878) (14.4802, 11.785) (14.6036, 11.646) (14.7117, 11.4947) (14.7965, 11.4043) (14.8447, 11.3653) (14.8975, 11.3328) (14.9531, 11.3055) (15.0111, 11.2836) (15.0914, 11.2644) (15.1942, 11.2519) (15.3182, 11.258) (15.4404, 11.2788) (15.5593, 11.3136) (15.6758, 11.3555) (15.788, 11.4079) (15.9348, 11.4834) (16.107, 11.5976) (16.3292, 11.7075) (16.557, 11.8044) (16.7895, 11.8894) (17.0253, 11.9646) (17.2638, 12.0308) (17.5044, 12.089) (17.7467, 12.1396) (17.9903, 12.1836) (18.1536, 12.2073) (18.2352, 12.2191) knots 0 0 0 0 0.024749 0.049497 0.074246 0.098994 0.123742 0.14849 0.173237 0.197983 0.222726 0.247472 0.259846 0.272219 0.284591 0.296962 0.309334 0.321703 0.334061 0.340251 0.346439 0.35262 0.358805 0.364993 0.371173 0.39592 0.420667 0.426846 0.433034 0.439219 0.4454 0.451589 0.457778 0.470137 0.482506 0.494877 0.507248 0.51962 0.531993 0.544367 0.569113 0.593856 0.618602 0.643349 0.668097 0.692845 0.717593 0.742342 0.767091 0.791839 0.791839 0.791839 0.791839
  spline S25 degree 3 poles (12.2191, 18.2352) (12.2073, 18.1536) (12.1836, 17.9903) (12.1396, 17.7467) (12.089, 17.5044) (12.0308, 17.2638) (11.9646, 17.0253) (11.8894, 16.7895) (11.8044, 16.557) (11.7075, 16.3292) (11.5976, 16.107) (11.4834, 15.9348) (11.4079, 15.788) (11.3555, 15.6758) (11.3136, 15.5593) (11.2788, 15.4404) (11.258, 15.3182) (11.2519, 15.1942) (11.2644, 15.0914) (11.2836, 15.0111) (11.3055, 14.9531) (11.3328, 14.8975) (11.3653, 14.8447) (11.4043, 14.7965) (11.4947, 14.7117) (11.646, 14.6036) (11.785, 14.4802) (11.8878, 14.4109) (11.9435, 14.3836) (12.0022, 14.3636) (12.0625, 14.3494) (12.1239, 14.341) (12.2065, 14.3401) (12.3095, 14.3508) (12.429, 14.3844) (12.5435, 14.4319) (12.6517, 14.4922) (12.7559, 14.559) (12.8537, 14.635) (12.98, 14.7414) (13.1225, 14.8909) (13.3146, 15.0476) (13.5151, 15.1927) (13.7229, 15.3273) (13.9361, 15.4531) (14.1539, 15.5708) (14.3755, 15.681) (14.6005, 15.7842) (14.8281, 15.8814) (14.9821, 15.9408) (15.059, 15.9705) knots 0 0 0 0 0.024749 0.049497 0.074246 0.098994 0.123742 0.14849 0.173237 0.197983 0.222726 0.247472 0.259846 0.272219 0.284591 0.296962 0.309334 0.321703 0.334061 0.340251 0.346439 0.35262 0.358805 0.364993 0.371173 0.39592 0.420667 0.426846 0.433034 0.439219 0.4454 0.451589 0.457778 0.470137 0.482506 0.494877 0.507248 0.51962 0.531993 0.544367 0.569113 0.593856 0.618602 0.643349 0.668097 0.692845 0.717593 0.742342 0.767091 0.791839 0.791839 0.791839 0.791839
  spline S26 degree 3 poles (7.855, 20.4971) (7.8617, 20.4148) (7.8749, 20.2504) (7.8862, 20.0031) (7.8908, 19.7556) (7.8876, 19.5081) (7.8761, 19.2608) (7.8553, 19.0142) (7.8242, 18.7686) (7.7804, 18.525) (7.7226, 18.2839) (7.6497, 18.0906) (7.6087, 17.9307) (7.5826, 17.8096) (7.5676, 17.6867) (7.5603, 17.563) (7.5672, 17.4393) (7.5887, 17.317) (7.6238, 17.2196) (7.6604, 17.1456) (7.6947, 17.0939) (7.7336, 17.0458) (7.7771, 17.0016) (7.8259, 16.9632) (7.9328, 16.9007) (8.1044, 16.829) (8.2674, 16.7395) (8.383, 16.6949) (8.4434, 16.6807) (8.5051, 16.6743) (8.567, 16.6738) (8.6288, 16.6792) (8.7095, 16.6967) (8.8075, 16.7301) (8.9165, 16.7894) (9.0176, 16.8612) (9.1097, 16.9441) (9.1964, 17.0325) (9.2748, 17.1283) (9.3743, 17.2601) (9.4799, 17.4376) (9.6324, 17.6331) (9.7956, 17.8192) (9.9682, 17.9967) (10.1481, 18.1667) (10.3342, 18.3299) (10.5257, 18.4867) (10.7221, 18.6374) (10.9224, 18.7828) (11.0593, 18.8749) (11.1277, 18.921) knots 0 0 0 0 0.024749 0.049497 0.074246 0.098994 0.123742 0.14849 0.173237 0.197983 0.222726 0.247472 0.259846 0.272219 0.284591 0.296962 0.309334 0.321703 0.334061 0.340251 0.346439 0.35262 0.358805 0.364993 0.371173 0.39592 0.420667 0.426846 0.433034 0.439219 0.4454 0.451589 0.457778 0.470137 0.482506 0.494877 0.507248 0.51962 0.531993 0.544367 0.569113 0.593856 0.618602 0.643349 0.668097 0.692845 0.717593 0.742342 0.767091 0.791839 0.791839 0.791839 0.791839
  spline S27 degree 3 poles (3.0971, 21.7311) (3.1218, 21.6524) (3.1714, 21.495) (3.2374, 21.2564) (3.297, 21.0162) (3.3489, 20.7742) (3.3927, 20.5305) (3.4273, 20.2854) (3.4516, 20.039) (3.4631, 19.7918) (3.4605, 19.5439) (3.4324, 19.3392) (3.428, 19.1742) (3.4295, 19.0504) (3.4422, 18.9272) (3.4626, 18.805) (3.4968, 18.6859) (3.5451, 18.5715) (3.6009, 18.4843) (3.6531, 18.4203) (3.698, 18.3775) (3.7467, 18.3393) (3.7989, 18.3059) (3.855, 18.2794) (3.9732, 18.2422) (4.1564, 18.2104) (4.3352, 18.1595) (4.4579, 18.1417) (4.5199, 18.1413) (4.5815, 18.1488) (4.6419, 18.1621) (4.701, 18.1811) (4.7757, 18.2162) (4.8639, 18.2705) (4.957, 18.3526) (5.0395, 18.4451) (5.1109, 18.5464) (5.1758, 18.6518) (5.2309, 18.7627) (5.2985, 18.9133) (5.362, 19.1099) (5.4672, 19.3344) (5.5848, 19.5521) (5.7136, 19.7636) (5.8512, 19.9694) (5.9963, 20.1699) (6.1481, 20.3654) (6.306, 20.556) (6.469, 20.7423) (6.5819, 20.8626) (6.6384, 20.9228) knots 0 0 0 0 0.024749 0.049497 0.074246 0.098994 0.123742 0.14849 0.173237 0.197983 0.222726 0.247472 0.259846 0.272219 0.284591 0.296962 0.309334 0.321703 0.334061 0.340251 0.346439 0.35262 0.358805 0.364993 0.371173 0.39592 0.420667 0.426846 0.433034 0.439219 0.4454 0.451589 0.457778 0.470137 0.482506 0.494877 0.507248 0.51962 0.531993 0.544367 0.569113 0.593856 0.618602 0.643349 0.668097 0.692845 0.717593 0.742342 0.767091 0.791839 0.791839 0.791839 0.791839
  circle A4 centre (0, 0) radius 2.5
  line L0 (2.5, 7) -> (2.5, -6.4701) construction
  line L1 (-2, 1.5) -> (-2, -1.5)
  point P0 (-1.6925, 21.661)
  point P1 (-1.5748, 21.4433)
  point P2 (-1.4634, 21.2223)
  point P3 (-1.359, 20.9979)
  point P4 (-1.2623, 20.7701)
  point P5 (-1.1742, 20.5389)
  point P6 (-1.0961, 20.304)
  point P7 (-1.0301, 20.0656)
  point P8 (-0.9804, 19.8232)
  point P9 (-0.9475, 19.5779)
  point P10 (-0.9238, 19.4564)
  point P11 (-0.8938, 19.3364)
  point P12 (-0.8546, 19.2191)
  point P13 (-0.8066, 19.105)
  point P14 (-0.7467, 18.9968)
  point P15 (-0.6737, 18.897)
  point P16 (-0.5858, 18.8101)
  point P17 (-0.5367, 18.7724)
  point P18 (-0.4836, 18.7405)
  point P19 (-0.4277, 18.7141)
  point P20 (-0.3694, 18.6935)
  point P21 (-0.309, 18.6803)
  point P22 (-0.2475, 18.6744)
  point P23 (0, 18.6744)
  point P24 (0.2475, 18.6744)
  point P25 (0.309, 18.6803)
  point P26 (0.3694, 18.6935)
  point P27 (0.4277, 18.7141)
  point P28 (0.4836, 18.7405)
  point P29 (0.5367, 18.7724)
  point P30 (0.5858, 18.8101)
  point P31 (0.6737, 18.897)
  point P32 (0.7467, 18.9968)
  point P33 (0.8066, 19.105)
  point P34 (0.8546, 19.2191)
  point P35 (0.8938, 19.3364)
  point P36 (0.9238, 19.4564)
  point P37 (0.9475, 19.5779)
  point P38 (0.9804, 19.8232)
  point P39 (1.0301, 20.0656)
  point P40 (1.0961, 20.304)
  point P41 (1.1742, 20.5389)
  point P42 (1.2623, 20.7701)
  point P43 (1.359, 20.9979)
  point P44 (1.4634, 21.2223)
  point P45 (1.5748, 21.4433)
  point P46 (1.6925, 21.661)
  point P47 (-5.8524, 19.9685)
  point P48 (-6.4701, 20.7413)
  point P49 (-5.7151, 19.7626)
  point P50 (-5.9974, 20.1691)
  point P51 (-5.5867, 19.5511)
  point P52 (-6.1491, 20.3646)
  point P53 (-5.4692, 19.3333)
  point P54 (-6.3069, 20.5553)
  point P55 (-5.3669, 19.108)
  point P56 (-5.2802, 18.8762)
  point P57 (-5.2301, 18.7631)
  point P58 (-5.1741, 18.6527)
  point P59 (-5.1098, 18.5471)
  point P60 (-5.0377, 18.4466)
  point P61 (-4.9552, 18.3543)
  point P62 (-4.8617, 18.2733)
  point P63 (-4.7567, 18.2081)
  point P64 (-4.7005, 18.1823)
  point P65 (-4.6417, 18.163)
  point P66 (-4.5813, 18.1497)
  point P67 (-4.458, 18.1432)
  point P68 (-4.3967, 18.1512)
  point P69 (-4.1554, 18.2062)
  point P70 (-4.5199, 18.1426)
  point P71 (-3.9142, 18.2613)
  point P72 (-3.8555, 18.2807)
  point P73 (-3.7995, 18.307)
  point P74 (-3.7473, 18.3401)
  point P75 (-3.6987, 18.3783)
  point P76 (-3.6541, 18.4212)
  point P77 (-3.6145, 18.4688)
  point P78 (-3.5482, 18.5731)
  point P79 (-3.4992, 18.6867)
  point P80 (-3.4649, 18.8055)
  point P81 (-3.4435, 18.9274)
  point P82 (-3.4314, 19.0505)
  point P83 (-3.4288, 19.1742)
  point P84 (-3.4328, 19.2979)
  point P85 (-3.4553, 19.5443)
  point P86 (-3.4495, 20.0389)
  point P87 (-3.4256, 20.2852)
  point P88 (-3.3912, 20.5303)
  point P89 (-3.3475, 20.7739)
  point P90 (-3.2957, 21.0159)
  point P91 (-3.2363, 21.2561)
  point P92 (-3.17, 21.4946)
  point P93 (-3.4608, 19.7917)
  point P94 (-10.1491, 18.1656)
  point P95 (-10.9232, 18.7816)
  point P96 (-9.9694, 17.9954)
  point P97 (-10.3351, 18.3288)
  point P98 (-9.7971, 17.8177)
  point P99 (-10.5265, 18.4857)
  point P100 (-9.6342, 17.6315)
  point P101 (-10.7227, 18.6365)
  point P102 (-9.4842, 17.4347)
  point P103 (-9.3482, 17.228)
  point P104 (-9.2742, 17.1288)
  point P105 (-9.195, 17.0337)
  point P106 (-9.1088, 16.945)
  point P107 (-9.0161, 16.8631)
  point P108 (-8.9152, 16.7915)
  point P109 (-8.806, 16.7333)
  point P110 (-8.6892, 16.6932)
  point P111 (-8.6286, 16.6805)
  point P112 (-8.5669, 16.6748)
  point P113 (-8.5051, 16.6753)
  point P114 (-8.3835, 16.6963)
  point P115 (-8.3255, 16.7177)
  point P116 (-8.1025, 16.825)
  point P117 (-8.4437, 16.682)
  point P118 (-7.8796, 16.9325)
  point P119 (-7.8267, 16.9644)
  point P120 (-7.778, 17.0026)
  point P121 (-7.7344, 17.0464)
  point P122 (-7.6955, 17.0945)
  point P123 (-7.6615, 17.1462)
  point P124 (-7.6336, 17.2015)
  point P125 (-7.5922, 17.3179)
  point P126 (-7.5696, 17.4395)
  point P127 (-7.5626, 17.563)
  point P128 (-7.5689, 17.6866)
  point P129 (-7.5845, 17.8093)
  point P130 (-7.6095, 17.9305)
  point P131 (-7.6409, 18.0502)
  point P132 (-7.7177, 18.2854)
  point P133 (-7.8221, 18.7689)
  point P134 (-7.8536, 19.0143)
  point P135 (-7.8745, 19.2609)
  point P136 (-7.8862, 19.5081)
  point P137 (-7.8895, 19.7556)
  point P138 (-7.8851, 20.003)
  point P139 (-7.8735, 20.2503)
  point P140 (-7.7781, 18.5254)
  point P141 (-13.9369, 15.4517)
  point P142 (-14.8287, 15.88)
  point P143 (-13.7238, 15.3258)
  point P144 (-14.1545, 15.5695)
  point P145 (-13.5163, 15.1909)
  point P146 (-14.376, 15.6799)
  point P147 (-13.316, 15.0457)
  point P148 (-14.6009, 15.7832)
  point P149 (-13.126, 14.8871)
  point P150 (-12.9474, 14.7159)
  point P151 (-12.8532, 14.6357)
  point P152 (-12.7548, 14.5606)
  point P153 (-12.651, 14.4933)
  point P154 (-12.5424, 14.434)
  point P155 (-12.4281, 14.3867)
  point P156 (-12.3088, 14.3543)
  point P157 (-12.1859, 14.3411)
  point P158 (-12.124, 14.3423)
  point P159 (-12.0626, 14.3504)
  point P160 (-12.0025, 14.3646)
  point P161 (-11.8885, 14.4122)
  point P162 (-11.8368, 14.446)
  point P163 (-11.6433, 14.6002)
  point P164 (-11.944, 14.3848)
  point P165 (-11.4498, 14.7546)
  point P166 (-11.4054, 14.7975)
  point P167 (-11.3664, 14.8455)
  point P168 (-11.3336, 14.898)
  point P169 (-11.3064, 14.9535)
  point P170 (-11.2848, 15.0115)
  point P171 (-11.2699, 15.0716)
  point P172 (-11.2554, 15.1943)
  point P173 (-11.2605, 15.3179)
  point P174 (-11.2812, 15.4398)
  point P175 (-11.3148, 15.5589)
  point P176 (-11.3573, 15.6751)
  point P177 (-11.4086, 15.7877)
  point P178 (-11.4659, 15.8974)
  point P179 (-11.5931, 16.1096)
  point P180 (-11.8024, 16.5577)
  point P181 (-11.8878, 16.79)
  point P182 (-11.9631, 17.0258)
  point P183 (-12.0295, 17.2642)
  point P184 (-12.0878, 17.5047)
  point P185 (-12.1385, 17.7469)
  point P186 (-12.1822, 17.9905)
  point P187 (-11.7053, 16.3301)
  point P188 (-17.0258, 11.9631)
  point P189 (-17.9905, 12.1822)
  point P190 (-16.79, 11.8878)
  point P191 (-17.2642, 12.0295)
  point P192 (-16.5577, 11.8024)
  point P193 (-17.5047, 12.0878)
  point P194 (-16.3301, 11.7053)
  point P195 (-17.7469, 12.1385)
  point P196 (-16.1096, 11.5931)
  point P197 (-15.8974, 11.4659)
  point P198 (-15.7877, 11.4086)
  point P199 (-15.6751, 11.3573)
  dimension "d4" = 360
  dimension "d6" = 5
  dimension "d7" = 4.5
  constraints: 4 centre point, 4 end point, 2 point on circle, 2 vertical, 1 coincident, 1 tangent, 2830 other
  measures "d6" diameter of A4
  measures "d7" distance between parallel lines of L0 L1
extrude "Выдавливание1" add sketch "Sketch1" against normal blind 6 contours S0 A3 S27 S26 S25 S24 S23 S22 S21 S20 S19 S18 S17 S16 S15 S14 S13 S12 S11 S10 S9 S8 S7 S6 S5 S4 S3 S2 S1 | L1 A4 picked at (-2.0912, -0.3466)
equation "\"d0\" = Ширина_грани"
equation "\"Модуль\" = 1.5"
equation "\"Угол_зацепления\" = 20deg"
equation "\"Зазор_профиля_зуба\" = 0.25"
equation "\"Радиус_закругления_зуба\" = 0.2386"
equation "\"Диаметр_головки\" = 43.90128"
equation "\"Диаметр_впадин\" = 37.34872"
equation "\"Основной_диаметр\" = 39.46709"
equation "\"Средний_диаметр\" = 42"
equation "\"Ширина_грани\" = 6"
equation "\"Коэффициент_смещения\" = -0.300426"
equation "\"Изменение_высоты_головки_зуба\" = 0.065814"
equation "\"Окружной_шаг\" = 4.71239"
equation "\"Общий_сдвиг_инструмента\" = -0.45064"
equation "\"Внутренний\" = 0"
